Autodesk Inventor part; units mm, degrees
(part 2 of 2)
  arc A581 (-20.3804, -2.2111) -> (-20.3335, -2.6078) centre (0, 0) ccw
  arc A582 (-20.1441, -3.8033) -> (-20.0662, -4.1951) centre (0, 0) ccw
  arc A583 (-19.7836, -5.372) -> (-19.6752, -5.7565) centre (0, 0) ccw
  arc A584 (-19.3011, -6.9077) -> (-19.1629, -7.2825) centre (0, 0) ccw
  arc A585 (-18.6997, -8.4007) -> (-18.5324, -8.7635) centre (0, 0) ccw
  arc A586 (-17.9829, -9.842) -> (-17.7877, -10.1905) centre (0, 0) ccw
  arc A587 (-17.1553, -11.2226) -> (-16.9334, -11.5547) centre (0, 0) ccw
  arc A588 (-16.2219, -12.534) -> (-15.9746, -12.8477) centre (0, 0) ccw
  arc A589 (-15.1885, -13.7681) -> (-14.9173, -14.0614) centre (0, 0) ccw
  arc A590 (-14.0614, -14.9173) -> (-13.7681, -15.1885) centre (0, 0) ccw
  arc A591 (-12.8477, -15.9746) -> (-12.534, -16.2219) centre (0, 0) ccw
  arc A592 (-11.5547, -16.9334) -> (-11.2226, -17.1553) centre (0, 0) ccw
  arc A593 (-10.1905, -17.7877) -> (-9.842, -17.9829) centre (0, 0) ccw
  arc A594 (-8.7635, -18.5324) -> (-8.4007, -18.6997) centre (0, 0) ccw
  arc A595 (-7.2825, -19.1629) -> (-6.9077, -19.3011) centre (0, 0) ccw
  arc A596 (-5.7565, -19.6752) -> (-5.372, -19.7836) centre (0, 0) ccw
  arc A597 (-4.1951, -20.0662) -> (-3.8033, -20.1441) centre (0, 0) ccw
  arc A598 (-2.6078, -20.3335) -> (-2.2111, -20.3804) centre (0, 0) ccw
  arc A599 (-1.0044, -20.4754) -> (-0.6052, -20.4911) centre (0, 0) ccw
  arc A600 (0.6052, -20.4911) -> (1.0044, -20.4754) centre (0, 0) ccw
  arc A601 (2.2111, -20.3804) -> (2.6078, -20.3335) centre (0, 0) ccw
  arc A602 (3.8033, -20.1441) -> (4.1951, -20.0662) centre (0, 0) ccw
  arc A603 (5.372, -19.7836) -> (5.7565, -19.6752) centre (0, 0) ccw
  arc A604 (6.9077, -19.3011) -> (7.2825, -19.1629) centre (0, 0) ccw
  arc A605 (8.4007, -18.6997) -> (8.7635, -18.5324) centre (0, 0) ccw
  arc A606 (9.842, -17.9829) -> (10.1905, -17.7877) centre (0, 0) ccw
  arc A607 (11.2226, -17.1553) -> (11.5547, -16.9334) centre (0, 0) ccw
  arc A608 (12.534, -16.2219) -> (12.8477, -15.9746) centre (0, 0) ccw
  arc A609 (13.7681, -15.1885) -> (14.0614, -14.9173) centre (0, 0) ccw
  arc A610 (14.9173, -14.0614) -> (15.1885, -13.7681) centre (0, 0) ccw
  arc A611 (15.9746, -12.8477) -> (16.2219, -12.534) centre (0, 0) ccw
  arc A612 (16.9334, -11.5547) -> (17.1553, -11.2226) centre (0, 0) ccw
  arc A613 (17.7877, -10.1905) -> (17.9829, -9.842) centre (0, 0) ccw
  arc A614 (18.5324, -8.7635) -> (18.6997, -8.4007) centre (0, 0) ccw
  arc A615 (19.1629, -7.2825) -> (19.3011, -6.9077) centre (0, 0) ccw
  arc A616 (19.6752, -5.7565) -> (19.7836, -5.372) centre (0, 0) ccw
  arc A617 (20.0662, -4.1951) -> (20.1441, -3.8033) centre (0, 0) ccw
  arc A618 (20.3335, -2.6078) -> (20.3804, -2.2111) centre (0, 0) ccw
  arc A619 (20.4754, -1.0044) -> (20.4911, -0.6052) centre (0, 0) ccw
  arc A620 (20.4911, 0.6052) -> (20.4754, 1.0044) centre (0, 0) ccw
  arc A621 (20.3804, 2.2111) -> (20.3335, 2.6078) centre (0, 0) ccw
  arc A622 (20.1441, 3.8033) -> (20.0662, 4.1951) centre (0, 0) ccw
  arc A623 (19.7836, 5.372) -> (19.6752, 5.7565) centre (0, 0) ccw
  arc A624 (19.3011, 6.9077) -> (19.1629, 7.2825) centre (0, 0) ccw
  arc A625 (18.6997, 8.4007) -> (18.5324, 8.7635) centre (0, 0) ccw
  arc A626 (17.9829, 9.842) -> (17.7877, 10.1905) centre (0, 0) ccw
  arc A627 (17.1553, 11.2226) -> (16.9334, 11.5547) centre (0, 0) ccw
  arc A628 (16.2219, 12.534) -> (15.9746, 12.8477) centre (0, 0) ccw
  arc A629 (15.1885, 13.7681) -> (14.9173, 14.0614) centre (0, 0) ccw
  arc A630 (14.0614, 14.9173) -> (13.7681, 15.1885) centre (0, 0) ccw
  arc A631 (12.8477, 15.9746) -> (12.534, 16.2219) centre (0, 0) ccw
  arc A632 (11.5547, 16.9334) -> (11.2226, 17.1553) centre (0, 0) ccw
  arc A633 (10.1905, 17.7877) -> (9.842, 17.9829) centre (0, 0) ccw
  arc A634 (8.7635, 18.5324) -> (8.4007, 18.6997) centre (0, 0) ccw
  arc A635 (7.2825, 19.1629) -> (6.9077, 19.3011) centre (0, 0) ccw
  arc A636 (5.7565, 19.6752) -> (5.372, 19.7836) centre (0, 0) ccw
  arc A637 (4.1951, 20.0662) -> (3.8033, 20.1441) centre (0, 0) ccw
  arc A638 (2.6078, 20.3335) -> (2.2111, 20.3804) centre (0, 0) ccw
  arc A639 (1.0044, 20.4754) -> (0.6052, 20.4911) centre (0, 0) ccw
  line L0 (-22.5, 0) -> (22.5, 0)
  line L1 (0, -22.5) -> (0, 22.5)
  circle A640 centre (0, 0) radius 20.5 projected
  point P0 (-0.9435, -3.4284)
  point P1 (-0.9435, -3.4284)
  constraints: 960 point on circle, 480 centre point, 4 end point, 2 horizontal alignment, 2 vertical alignment, 1 vertical, 2082 other
extrude "押し出し1" cut sketch "スケッチ4" against normal blind 10 contours A0 A480 L1 A640 A2 A1 | A480 A240 A241 A242 A640 L1 | A640 A239 A238 A237 A559 A477 A478 A479 | L0 A640 A62 A61 A60 A500 | A500 A300 A301 A302 A640 L0 | L0 A640 A182 A181 A180 A540 | A540 A420 A421 A422 A640 L0 | L1 A640 A122 A121 A120 A520 | A520 A360 A361 A362 A640 L1 | A5 A4 A3 A481 A243 A244 A245 A640 | A640 A236 A235 A234 A558 A474 A475 A476 | A640 A59 A58 A57 A499 A297 A298 A299 | A65 A64 A63 A501 A303 A304 A305 A640 | A185 A184 A183 A541 A423 A424 A425 A640 | A640 A179 A178 A177 A539 A417 A418 A419 | A640 A119 A118 A117 A519 A357 A358 A359 | A125 A124 A123 A521 A363 A364 A365 A640 | A8 A7 A6 A482 A246 A247 A248 A640 | A640 A233 A232 A231 A557 A471 A472 A473 | A640 A56 A55 A54 A498 A294 A295 A296 | A68 A67 A66 A502 A306 A307 A308 A640 | A188 A187 A186 A542 A426 A427 A428 A640 | A640 A176 A175 A174 A538 A414 A415 A416 | A640 A116 A115 A114 A518 A354 A355 A356 | A128 A127 A126 A522 A366 A367 A368 A640 | A11 A10 A9 A483 A249 A250 A251 A640 | A640 A230 A229 A228 A556 A468 A469 A470 | A640 A53 A52 A51 A497 A291 A292 A293 | A71 A70 A69 A503 A309 A310 A311 A640 | A191 A190 A189 A543 A429 A430 A431 A640 | A640 A173 A172 A171 A537 A411 A412 A413 | A640 A113 A112 A111 A517 A351 A352 A353 | A131 A130 A129 A523 A369 A370 A371 A640 | A14 A13 A12 A484 A252 A253 A254 A640 | A640 A227 A226 A225 A555 A465 A466 A467 | A640 A50 A49 A48 A496 A288 A289 A290 | A74 A73 A72 A504 A312 A313 A314 A640 | A194 A193 A192 A544 A432 A433 A434 A640 | A640 A170 A169 A168 A536 A408 A409 A410 | A640 A110 A109 A108 A516 A348 A349 A350 | A134 A133 A132 A524 A372 A373 A374 A640 | A17 A16 A15 A485 A255 A256 A257 A640 | A640 A224 A223 A222 A554 A462 A463 A464 | A640 A47 A46 A45 A495 A285 A286 A287 | A77 A76 A75 A505 A315 A316 A317 A640 | A197 A196 A195 A545 A435 A436 A437 A640 | A640 A167 A166 A165 A535 A405 A406 A407 | A640 A107 A106 A105 A515 A345 A346 A347 | A137 A136 A135 A525 A375 A376 A377 A640 | A20 A19 A18 A486 A258 A259 A260 A640 | A640 A221 A220 A219 A553 A459 A460 A461 | A640 A44 A43 A42 A494 A282 A283 A284 | A80 A79 A78 A506 A318 A319 A320 A640 | A200 A199 A198 A546 A438 A439 A440 A640 | A640 A164 A163 A162 A534 A402 A403 A404 | A640 A104 A103 A102 A514 A342 A343 A344 | A140 A139 A138 A526 A378 A379 A380 A640 | A23 A22 A21 A487 A261 A262 A263 A640 | A640 A218 A217 A216 A552 A456 A457 A458 | A640 A41 A40 A39 A493 A279 A280 A281 | A83 A82 A81 A507 A321 A322 A323 A640 | A203 A202 A201 A547 A441 A442 A443 A640 | A640 A161 A160 A159 A533 A399 A400 A401 | A640 A101 A100 A99 A513 A339 A340 A341 | A143 A142 A141 A527 A381 A382 A383 A640 | A26 A25 A24 A488 A264 A265 A266 A640 | A640 A215 A214 A213 A551 A453 A454 A455 | A640 A38 A37 A36 A492 A276 A277 A278 | A86 A85 A84 A508 A324 A325 A326 A640 | A206 A205 A204 A548 A444 A445 A446 A640 | A640 A158 A157 A156 A532 A396 A397 A398 | A640 A98 A97 A96 A512 A336 A337 A338 | A146 A145 A144 A528 A384 A385 A386 A640 | A29 A28 A27 A489 A267 A268 A269 A640 | A640 A212 A211 A210 A550 A450 A451 A452 | A640 A35 A34 A33 A491 A273 A274 A275 | A89 A88 A87 A509 A327 A328 A329 A640 | A209 A208 A207 A549 A447 A448 A449 A640 | A640 A155 A154 A153 A531 A393 A394 A395 | A640 A95 A94 A93 A511 A333 A334 A335 | A149 A148 A147 A529 A387 A388 A389 A640 | A32 A31 A30 A490 A270 A271 A272 A640 | A92 A91 A90 A510 A330 A331 A332 A640 | A640 A152 A151 A150 A530 A390 A391 A392
body "Solid1"
